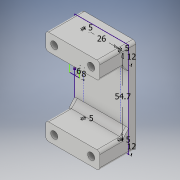
# Autodesk Inventor part: MotorClamp
Saved by Autodesk Inventor 2018 (Build 220112000, 112)
## iProperties
Created: 2017-08-07
Part Number: MotorClamp
Material: Generic
Document SubType Name: Modeling
Designer: Akram Al-Hourani
Density: 1 g/cm^3
Appearance: Default
Author: Akram Al-Hourani
Autodesk Inventor part; units mm, degrees
ref_plane "YZ Plane" through (0, 0, 0) normal (1, 0, 0) x (0, 1, 0)
ref_plane "XZ Plane" through (0, 0, 0) normal (0, 1, 0) x (-1, 0, 0)
ref_plane "XY Plane" through (0, 0, 0) normal (0, 0, 1) x (1, 0, 0)
sketch "Sketch1" plane through (0, 0, 0) normal (0, 0, 1) x (1, 0, 0)
  line L0 (0, 0) -> (26, 0) construction
  line L1 (26, 0) -> (26, 54.7) construction
  line L2 (26, 54.7) -> (0, 54.7) construction
  line L3 (0, 54.7) -> (0, 0) construction
  circle A0 centre (0, 54.7) radius 2.5
  circle A1 centre (26, 54.7) radius 2.5
  circle A2 centre (26, 0) radius 2.5
  circle A3 centre (0, 0) radius 2.5
  line L4 (-6, -6) -> (32, -6)
  line L5 (32, -6) -> (32, 60.7)
  line L6 (32, 60.7) -> (-6, 60.7)
  line L7 (-6, 60.7) -> (-6, -6)
  line L8 (-6, -6) -> (32, -6)
  line L9 (32, -6) -> (32, 6)
  line L10 (32, 6) -> (-6, 6)
  line L11 (-6, 6) -> (-6, -6)
  line L12 (-6, 60.7) -> (32, 60.7)
  line L13 (32, 60.7) -> (32, 48.7)
  line L14 (32, 48.7) -> (-6, 48.7)
  line L15 (-6, 48.7) -> (-6, 60.7)
  line L16 (32, 48.7) -> (-6, 48.7)
  line L17 (-6, 48.7) -> (-6, 6)
  line L18 (-6, 6) -> (32, 6)
  line L19 (32, 6) -> (32, 48.7)
  line L20 (-6, 60.7) -> (32, 60.7)
  line L21 (32, 60.7) -> (32, 48.7)
  line L22 (32, 48.7) -> (-6, 48.7)
  line L23 (-6, 48.7) -> (-6, 60.7)
  line L24 (-6, 6) -> (32, 6)
  line L25 (32, 6) -> (32, -6)
  line L26 (32, -6) -> (-6, -6)
  line L27 (-6, -6) -> (-6, 6)
  line L28 (-9.5, 23.35) -> (-2.5, 23.35)
  line L29 (-2.5, 23.35) -> (-2.5, 31.35)
  line L30 (-2.5, 31.35) -> (-9.5, 31.35)
  line L31 (-9.5, 31.35) -> (-9.5, 23.35)
  line L32 (-9.5, 23.35) -> (-2.5, 31.35) construction
  line L33 (-2.5, 23.35) -> (-9.5, 31.35) construction
  point P0 (-6, 27.35)
  dimension "d0" = 26
  dimension "d1" = 54.7
  dimension "d2" = 5
  dimension "d3" = 5
  dimension "d4" = 5
  dimension "d5" = 5
  dimension "d6" = 6
  dimension "d7" = 12
  dimension "d8" = 12
  dimension "d23" = 8
  constraints: 68 end point, 16 parallel, 8 perpendicular, 7 horizontal, 4 centre point, 4 coincident, 3 midpoint, 2 point on line, 3 other
  measures "d0" distance of L2.end L1.end
  measures "d1" distance of L1.end L0.end
  measures "d2" diameter of A0
  measures "d3" diameter of A1
  measures "d4" diameter of A2
  measures "d5" diameter of A3
  measures "d6" distance between parallel lines of L3 L7
  measures "d7" distance of L9.end L8.end
  measures "d8" distance of L12.end L13.end
  measures "d23" distance of L29.end L28.end
extrude "Extrusion1" add sketch "Sketch1" against normal blind 5 contours A0 | A1 | A2 | A3 | L7 L10 L5 L4 | L7 L28 L29 L30 L14 L5 L10 | L7 L30 L29 L28 | L14 L7 L6 L5
extrude "Extrusion2" add sketch "Sketch1" along normal blind 20.3 contours L14 L7 L6 L5
extrude "Extrusion3" add sketch "Sketch1" along normal blind 20.3 contours L7 L10 L5 L4
extrude "Extrusion4" cut sketch "Sketch1" against normal blind 5 contours A2 | A3
extrude "Extrusion5" cut sketch "Sketch1" against normal blind 5 contours A0 | A1
fillet "Fillet1" radius 2 8 edges at (32, 48.7, 10.15) (-6, 48.7, 10.15) (32, 6, 10.15) (-6, 6, 10.15) (32, -6, 7.65) (-6, -6, 7.65) (-6, 60.7, 7.65) (32, 60.7, 7.65)
chamfer "Chamfer1" distance 4.2 angle 45 6 edges at (13, 48.7, 0) (-5.4142, 49.2858, 0) (31.4142, 49.2858, 0) (13, 6, 0) (31.4142, 5.4142, 0) (-5.4142, 5.4142, 0)
extrude "Extrusion6" cut sketch "Sketch1" against normal blind 5 contours L28 L31 L30 L7 | L7 L30 L29 L28
equation "\"d15\" = d3"
equation "\"d17\" = d3"
equation "\"d24\" = d3"
body "Solid1"
